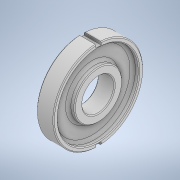
# Autodesk Inventor part: Тихоходное колесо
Saved by Autodesk Inventor 2021 (Build 250183000, 183)
## iProperties
Created: 2023-05-08
Part Number: Тихоходное колесо
Material: Типовые
Document SubType Name: Modeling
Designer: gdevc
Density: 1 g/cm^3
Appearance: По умолчанию
Author: gdevc
Autodesk Inventor part; units mm, degrees
ref_plane "YZ Plane" through (0, 0, 0) normal (1, 0, 0) x (0, 1, 0)
ref_plane "XZ Plane" through (0, 0, 0) normal (0, 1, 0) x (-1, 0, 0)
ref_plane "XY Plane" through (0, 0, 0) normal (0, 0, 1) x (1, 0, 0)
sketch "Эскиз1" plane through (0, 0, 0) normal (0, 0, 1) x (1, 0, 0)
  line L0 (0, 0) -> (28.5418, 0) construction
  line L1 (0, 30) -> (32, 30)
  line L2 (32, 30) -> (32, 45)
  line L3 (32, 45) -> (25, 45)
  line L4 (20, 50) -> (20, 71.15)
  line L5 (25, 76.15) -> (32, 76.15)
  line L6 (32, 76.15) -> (32, 84.358)
  line L7 (32, 84.358) -> (9.7618, 84.358)
  line L8 (9.7618, 84.358) -> (0, 84.358)
  line L9 (0, 84.358) -> (0, 76.15)
  line L10 (0, 76.15) -> (7, 76.15)
  line L11 (12, 71.15) -> (12, 50)
  line L12 (7, 45) -> (0, 45)
  line L13 (0, 45) -> (0, 30)
  arc A0 (7, 45) -> (12, 50) centre (7, 50) ccw
  arc A1 (12, 71.15) -> (7, 76.15) centre (7, 71.15) ccw
  arc A2 (25, 76.15) -> (20, 71.15) centre (25, 71.15) ccw
  arc A3 (20, 50) -> (25, 45) centre (25, 50) ccw
  point P0 (11, 45)
  point P1 (12, 46)
  point P2 (21, 45)
  point P3 (20, 46)
  point P4 (12, 75.15)
  point P5 (11, 76.15)
  point P6 (21, 76.15)
  point P7 (20, 75.15)
  dimension "d0" = 32
  dimension "d3" = 32
  dimension "d7" = 60
  dimension "d8" = 168.716
  dimension "d10" = 152.3
  dimension "d11" = 90
  dimension "d12" = 152.3
  dimension "d13" = 90
  dimension "d15" = 8
  dimension "d16" = 12
  dimension "d23" = 5
  constraints: 28 end point, 11 point on line, 9 perpendicular, 8 point on circle, 8 tangent, 4 centre point, 3 equal radius, 3 horizontal, 1 vertical
  measures "d0" distance of L1.start L1.end
  measures "d3" distance between parallel lines of L6 L9
  measures "d7" diameter of L1 L0
  measures "d8" diameter of L7 L0
  measures "d10" diameter of L10 L0
  measures "d11" diameter of L12 L0
  measures "d12" diameter of L5 L0
  measures "d13" diameter of L3 L0
  measures "d15" distance between parallel lines of L4 L11
  measures "d16" distance between parallel lines of L13 L11
  measures "d23" radius of A0
revolve "Вращение1" add sketch "Эскиз1" angle 360 about axis through (0, 0, 0) along (1, 0, 0)
chamfer "Фаска1" distance 1.6 angle 45 8 edges at (0, -84.358, 0) (0, -76.15, 0) (32, -84.358, 0) (32, -76.15, 0) (32, -30, 0) (0, -30, 0) (32, -45, 0) (0, -45, 0)
sketch "Эскиз3" plane through (0, 0, 0) normal (0, 0, 1) x (1, 0, 0)
  line L0 (1.6, 84.358) -> (30.4, 84.358) projected
  line L1 (7, 76.15) -> (1.6, 76.15) projected
  line L2 (0, -82.758) -> (0, 82.758) projected
  line L3 (32, 82.758) -> (32, -82.758) projected
  line L4 (1.6, 84.358) -> (37.8818, 84.358)
  line L5 (37.8818, 84.358) -> (37.8818, 78.608)
  line L6 (37.8818, 78.608) -> (1.6, 78.608)
  line L7 (1.6, 78.608) -> (-1.0807, 78.608)
  line L8 (-1.0807, 78.608) -> (-1.0807, 84.358)
  line L9 (-1.0807, 84.358) -> (2.0712, 84.358)
  line L10 (0, 0) -> (69.5045, 0)
  line L11 (1.6, -84.358) -> (30.4, -84.358)
  line L12 (7, -76.15) -> (1.6, -76.15)
  line L13 (1.6, -84.358) -> (37.8818, -84.358)
  line L14 (37.8818, -84.358) -> (37.8818, -78.608)
  line L15 (37.8818, -78.608) -> (1.6, -78.608)
  line L16 (1.6, -78.608) -> (-1.0807, -78.608)
  line L17 (-1.0807, -78.608) -> (-1.0807, -84.358)
  line L18 (-1.0807, -84.358) -> (2.0712, -84.358)
  dimension "d20" = 78.608
  constraints: 30 end point, 10 symmetric about line, 3 horizontal, 2 perpendicular, 2 point on line, 1 parallel
  measures "d20" distance from line of L10.start L6
extrude "Выдавливание1" cut sketch "Эскиз3" against normal mid plane 10 contours L0 L4 L5 L6 L7 L8 L9 | L16 L15 L14 L13 L11 L18 L17
equation "\"d16\" = -0.5 * d15 + 0.5 * d0"
